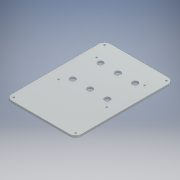
# Autodesk Inventor part: BackPanel
Saved by Autodesk Inventor 2016 (Build 200138000, 138)
## iProperties
Created: 2015-09-18
Part Number: BackPanel
Material: Generic
Document SubType Name: Modeling
Designer: Erin
Density: 1 g/cm^3
Appearance: Default
Author: Erin
Autodesk Inventor part; units mm, degrees
ref_plane "YZ Plane" through (0, 0, 0) normal (1, 0, 0) x (0, 1, 0)
ref_plane "XZ Plane" through (0, 0, 0) normal (0, 1, 0) x (-1, 0, 0)
ref_plane "XY Plane" through (0, 0, 0) normal (0, 0, 1) x (1, 0, 0)
derived "FrontPanel.ipt"
sketch "Sketch1" plane through (0, 0, 0) normal (0, 0, 1) x (1, 0, 0)
  line L0 (-60, 85) -> (60, 85)
  line L1 (60, 85) -> (60, -85)
  line L2 (60, -85) -> (-60, -85)
  line L3 (-60, -85) -> (-60, 85)
  line L4 (-50, 56.6301) -> (50, 56.6301)
  line L5 (50, 56.6301) -> (50, -13.3699)
  line L6 (50, -13.3699) -> (-50, -13.3699)
  line L7 (-50, -13.3699) -> (-50, 56.6301)
  circle A0 centre (-25, -55) radius 13.85
  circle A1 centre (-25, -24.425) radius 2.7
  circle A2 centre (25, -24.425) radius 2.7
  line L8 (-25, 85) -> (-25, -85) construction
  line L9 (-60, -55) -> (60, -55) construction
  circle A3 centre (-25, -55) radius 17.875 construction
  line L10 (25, 85) -> (25, -85) construction
  circle A4 centre (25, -55) radius 13.85
  circle A5 centre (25, -55) radius 17.875 construction
  circle A6 centre (-53.4, -78.4) radius 1.6
  line L11 (-52.9471, 75) -> (52.9471, 75) construction
  line L12 (52.9471, 75) -> (52.9471, 66.6301) construction
  line L13 (52.9471, 66.6301) -> (-52.9471, 66.6301) construction
  line L14 (-52.9471, 66.6301) -> (-52.9471, 75) construction
  circle A7 centre (-43.4, -6.7699) radius 1.6
  line L15 (-50, 21.6301) -> (50, 21.6301) construction
  line L16 (0, 56.6301) -> (0, -13.3699) construction
  circle A8 centre (-43.4, 50.0301) radius 1.6
  circle A9 centre (43.4, 50.0301) radius 1.6
  circle A10 centre (43.4, -6.7699) radius 1.6
  line L17 (-60, 0) -> (60, 0) construction
  circle A11 centre (53.4, -78.4) radius 1.6
  circle A12 centre (53.4, 78.4) radius 1.6
  circle A13 centre (-53.4, 78.4) radius 1.6
  point P0 (0, 0)
  point P1 (0, 85)
  point P2 (0, 75)
extrude "Extrusion1" add sketch "Sketch1" along normal blind 3 contours L0 L1 L2 L3 | L4 L5 L6 L7 | A0 | A1 | A2 | A4 | A7 | A8 | A9 | A10
fillet "Fillet1" radius 10 4 edges at (-60, -85, 1.5) (60, -85, 1.5) (60, 85, 1.5) (-60, 85, 1.5)
sketch "Sketch2" plane through (-50, -85, 3) normal (0, 0, 1) x (1, 0, 0)
  arc A0 (0, 170) -> (-10, 160) centre (0, 160) ccw projected
  line L0 (-10, 160) -> (-10, 10) projected
  arc A1 (-10, 10) -> (0, 0) centre (0, 10) ccw projected
  line L1 (0, 0) -> (100, 0) projected
  arc A2 (100, 0) -> (110, 10) centre (100, 10) ccw projected
  line L2 (110, 10) -> (110, 160) projected
  arc A3 (110, 160) -> (100, 170) centre (100, 160) ccw projected
  line L3 (100, 170) -> (0, 170) projected
  circle A4 centre (103.4, 6.6) radius 1.6 projected
  circle A5 centre (103.4, 163.4) radius 1.6 projected
  circle A6 centre (-3.4, 163.4) radius 1.6 projected
  circle A7 centre (-3.4, 6.6) radius 1.6 projected
  circle A8 centre (20.0375, 132.9625) radius 4.9625
  line L4 (-10, 85) -> (110, 85) construction
  line L5 (100, 170) -> (0, 170) projected
  line L6 (50, 170) -> (50, 0) construction
  line L7 (0, 0) -> (100, 0) projected
  circle A9 centre (50, 132.9625) radius 4.9625
  circle A10 centre (20.0375, 85) radius 4.9625
  circle A11 centre (50, 85) radius 4.9625
  line L8 (5, 140) -> (95, 140)
  line L9 (95, 140) -> (95, 70)
  line L10 (95, 70) -> (5, 70)
  line L11 (5, 70) -> (5, 140)
  circle A12 centre (8.5083, 72.2583) radius 1.5083
  line L12 (5, 105) -> (95, 105) construction
  circle A13 centre (8.5083, 137.7417) radius 1.5083
  circle A14 centre (91.4917, 72.2583) radius 1.5083
  circle A15 centre (91.4917, 137.7417) radius 1.5083
  point P0 (50, 140)
  dimension "d4" = 9.925
  dimension "d5" = 25
  dimension "d6" = 43
  dimension "d7" = 9.925
  dimension "d8" = 9.925
  dimension "d9" = 9.925
  dimension "d14" = 43
  dimension "d15" = 90
  dimension "d16" = 70
  dimension "d17" = 30
  dimension "d18" = 3.0167
  dimension "d19" = 0.75
  dimension "d20" = 2
  constraints: 14 end point, 8 centre point, 8 midpoint, 3 symmetric about line, 2 parallel, 2 point on line, 1 coincident, 1 horizontal, 1 perpendicular, 1 vertical alignment, 3 other
  measures "d4" diameter of A8
  measures "d5" distance edge to line of A8 L6
  measures "d6" distance edge to line of A8 L4
  measures "d7" diameter of A9
  measures "d8" diameter of A10
  measures "d9" diameter of A11
  measures "d14" distance edge to line of A9 L4
  measures "d15" distance of L9.end L10.end
  measures "d16" distance of L8.end L9.end
  measures "d17" distance between parallel lines of L8 L3
  measures "d18" diameter of A12
  measures "d19" distance edge to line of A12 L10
  measures "d20" distance edge to line of A12 L11
extrude "Extrusion2" cut sketch "Sketch2" against normal blind 3 contours A8 | A10
extrude "Extrusion3" cut sketch "Sketch2" against normal blind 3 contours A9 | A11
mirror "Mirror1" about plane through (0, 0, 0) normal (1, 0, 0) of "Extrusion2"
extrude "Extrusion4" cut sketch "Sketch2" against normal blind 3 contours A12 | A13 | A14 | A15
equation "\"d18\" = m3 + 0.0416667 * k"
equation "\"m3\" = 3"
equation "\"k\" = 0.4"
body "Solid1"
